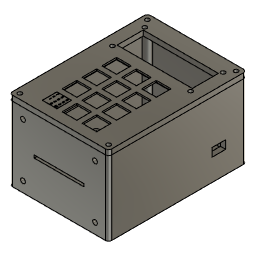
BinaryInterfacer v13 (Autodesk Fusion 360 design; units mm, degrees)
Autodesk Fusion 360 part; units mm, degrees
(part 1 of 2)
sketch "Sketch1" plane through (0, 0, 0) normal (0, 0, 1) x (1, 0, 0) in component "Plate"
  line L0 (6.725, 7.025) -> (-6.725, 7.025)
  line L1 (-7.025, 6.725) -> (-7.025, -6.725)
  line L2 (-6.725, -7.025) -> (6.725, -7.025)
  line L3 (7.025, -6.725) -> (7.025, 6.725)
  line L4 (7.025, 7.025) -> (-7.025, -7.025) construction
  line L5 (-7.025, 7.025) -> (7.025, -7.025) construction
  arc A0 (-6.725, 7.025) -> (-7.025, 6.725) centre (-6.725, 6.725) ccw
  arc A1 (-7.025, -6.725) -> (-6.725, -7.025) centre (-6.725, -6.725) ccw
  arc A2 (6.725, -7.025) -> (7.025, -6.725) centre (6.725, -6.725) ccw
  arc A3 (7.025, 6.725) -> (6.725, 7.025) centre (6.725, 6.725) ccw
  line L6 (26.075, -6.725) -> (26.075, 6.725)
  arc A4 (26.075, 6.725) -> (25.775, 7.025) centre (25.775, 6.725) ccw
  line L7 (25.775, 7.025) -> (12.325, 7.025)
  arc A5 (12.325, 7.025) -> (12.025, 6.725) centre (12.325, 6.725) ccw
  line L8 (12.025, 6.725) -> (12.025, -6.725)
  arc A6 (12.025, -6.725) -> (12.325, -7.025) centre (12.325, -6.725) ccw
  line L9 (12.325, -7.025) -> (25.775, -7.025)
  arc A7 (25.775, -7.025) -> (26.075, -6.725) centre (25.775, -6.725) ccw
  line L10 (45.125, -6.725) -> (45.125, 6.725)
  arc A8 (45.125, 6.725) -> (44.825, 7.025) centre (44.825, 6.725) ccw
  line L11 (44.825, 7.025) -> (31.375, 7.025)
  arc A9 (31.375, 7.025) -> (31.075, 6.725) centre (31.375, 6.725) ccw
  line L12 (31.075, 6.725) -> (31.075, -6.725)
  arc A10 (31.075, -6.725) -> (31.375, -7.025) centre (31.375, -6.725) ccw
  line L13 (31.375, -7.025) -> (44.825, -7.025)
  arc A11 (44.825, -7.025) -> (45.125, -6.725) centre (44.825, -6.725) ccw
  line L14 (7.025, 12.325) -> (7.025, 25.775)
  arc A12 (7.025, 25.775) -> (6.725, 26.075) centre (6.725, 25.775) ccw
  line L15 (6.725, 26.075) -> (-6.725, 26.075)
  arc A13 (-6.725, 26.075) -> (-7.025, 25.775) centre (-6.725, 25.775) ccw
  line L16 (-7.025, 25.775) -> (-7.025, 12.325)
  arc A14 (-7.025, 12.325) -> (-6.725, 12.025) centre (-6.725, 12.325) ccw
  line L17 (-6.725, 12.025) -> (6.725, 12.025)
  arc A15 (6.725, 12.025) -> (7.025, 12.325) centre (6.725, 12.325) ccw
  line L18 (26.075, 12.325) -> (26.075, 25.775)
  arc A16 (26.075, 25.775) -> (25.775, 26.075) centre (25.775, 25.775) ccw
  line L19 (25.775, 26.075) -> (12.325, 26.075)
  arc A17 (12.325, 26.075) -> (12.025, 25.775) centre (12.325, 25.775) ccw
  line L20 (12.025, 25.775) -> (12.025, 12.325)
  arc A18 (12.025, 12.325) -> (12.325, 12.025) centre (12.325, 12.325) ccw
  line L21 (12.325, 12.025) -> (25.775, 12.025)
  arc A19 (25.775, 12.025) -> (26.075, 12.325) centre (25.775, 12.325) ccw
  line L22 (45.125, 12.325) -> (45.125, 25.775)
  arc A20 (45.125, 25.775) -> (44.825, 26.075) centre (44.825, 25.775) ccw
  line L23 (44.825, 26.075) -> (31.375, 26.075)
  arc A21 (31.375, 26.075) -> (31.075, 25.775) centre (31.375, 25.775) ccw
  line L24 (31.075, 25.775) -> (31.075, 12.325)
  arc A22 (31.075, 12.325) -> (31.375, 12.025) centre (31.375, 12.325) ccw
  line L25 (31.375, 12.025) -> (44.825, 12.025)
  arc A23 (44.825, 12.025) -> (45.125, 12.325) centre (44.825, 12.325) ccw
  line L26 (7.025, 31.375) -> (7.025, 44.825)
  arc A24 (7.025, 44.825) -> (6.725, 45.125) centre (6.725, 44.825) ccw
  line L27 (6.725, 45.125) -> (-6.725, 45.125)
  arc A25 (-6.725, 45.125) -> (-7.025, 44.825) centre (-6.725, 44.825) ccw
  line L28 (-7.025, 44.825) -> (-7.025, 31.375)
  arc A26 (-7.025, 31.375) -> (-6.725, 31.075) centre (-6.725, 31.375) ccw
  line L29 (-6.725, 31.075) -> (6.725, 31.075)
  arc A27 (6.725, 31.075) -> (7.025, 31.375) centre (6.725, 31.375) ccw
  line L30 (26.075, 31.375) -> (26.075, 44.825)
  arc A28 (26.075, 44.825) -> (25.775, 45.125) centre (25.775, 44.825) ccw
  line L31 (25.775, 45.125) -> (12.325, 45.125)
  arc A29 (12.325, 45.125) -> (12.025, 44.825) centre (12.325, 44.825) ccw
  line L32 (12.025, 44.825) -> (12.025, 31.375)
  arc A30 (12.025, 31.375) -> (12.325, 31.075) centre (12.325, 31.375) ccw
  line L33 (12.325, 31.075) -> (25.775, 31.075)
  arc A31 (25.775, 31.075) -> (26.075, 31.375) centre (25.775, 31.375) ccw
  line L34 (45.125, 31.375) -> (45.125, 44.825)
  arc A32 (45.125, 44.825) -> (44.825, 45.125) centre (44.825, 44.825) ccw
  line L35 (44.825, 45.125) -> (31.375, 45.125)
  arc A33 (31.375, 45.125) -> (31.075, 44.825) centre (31.375, 44.825) ccw
  line L36 (31.075, 44.825) -> (31.075, 31.375)
  arc A34 (31.075, 31.375) -> (31.375, 31.075) centre (31.375, 31.375) ccw
  line L37 (31.375, 31.075) -> (44.825, 31.075)
  arc A35 (44.825, 31.075) -> (45.125, 31.375) centre (44.825, 31.375) ccw
  arc A36 (12.025, -25.775) -> (12.325, -26.075) centre (12.325, -25.775) ccw
  arc A37 (25.775, -26.075) -> (26.075, -25.775) centre (25.775, -25.775) ccw
  arc A38 (26.075, -12.325) -> (25.775, -12.025) centre (25.775, -12.325) ccw
  arc A39 (12.325, -12.025) -> (12.025, -12.325) centre (12.325, -12.325) ccw
  line L38 (12.325, -26.075) -> (25.775, -26.075)
  line L39 (26.075, -25.775) -> (26.075, -12.325)
  line L40 (12.025, -12.325) -> (12.025, -25.775)
  line L41 (25.775, -12.025) -> (12.325, -12.025)
  line L42 (-28.45, 96.125) -> (66.55, 96.125)
  line L43 (66.55, 96.125) -> (66.55, -36.075)
  line L44 (66.55, -36.075) -> (-28.45, -36.075)
  line L45 (-28.45, -36.075) -> (-28.45, 96.125)
  line L46 (26.075, -19.05) -> (66.55, -19.05) construction
  line L47 (12.025, -19.05) -> (-28.45, -19.05) construction
  line L48 (19.05, 96.125) -> (19.05, -36.075) construction
  line L49 (59.05, 50.125) -> (-20.95, 50.125)
  line L50 (-20.95, 50.125) -> (-20.95, 86.125)
  line L51 (-20.95, 86.125) -> (59.05, 86.125)
  line L52 (59.05, 86.125) -> (59.05, 50.125)
  line L53 (59.05, 50.125) -> (-20.95, 86.125) construction
  line L54 (-20.95, 50.125) -> (59.05, 86.125) construction
  line L55 (-16.95, 80.625) -> (55.05, 80.625)
  line L56 (55.05, 80.625) -> (55.05, 55.625)
  line L57 (55.05, 55.625) -> (-16.95, 55.625)
  line L58 (-16.95, 55.625) -> (-16.95, 80.625)
  line L59 (-16.95, 80.625) -> (55.05, 55.625) construction
  line L60 (55.05, 80.625) -> (-16.95, 55.625) construction
  line L61 (-18.45, 86.125) -> (-18.45, 50.125) construction
  line L62 (56.55, 86.125) -> (56.55, 50.125) construction
  line L63 (-18.45, 68.125) -> (-20.95, 68.125) construction
  line L64 (56.55, 68.125) -> (59.05, 68.125) construction
  circle A40 centre (-18.45, 83.625) radius 2
  circle A41 centre (-18.45, 52.625) radius 2
  circle A42 centre (56.55, 83.625) radius 2
  circle A43 centre (56.55, 52.625) radius 2
  circle A44 centre (-23.45, -31.075) radius 5 construction
  circle A45 centre (-23.45, -31.075) radius 2
  circle A46 centre (61.55, -31.075) radius 2
  line L65 (19.05, 30.025) -> (23, 30.025) construction
  circle A47 centre (-23.45, 91.125) radius 2
  circle A48 centre (61.55, 91.125) radius 2
  line L66 (-10.025, 48.125) -> (48.125, 48.125)
  line L67 (48.125, 48.125) -> (48.125, -29.075)
  line L68 (48.125, -29.075) -> (-10.025, -29.075)
  line L69 (-10.025, -29.075) -> (-10.025, 48.125)
  line L70 (-7.025, 38.1) -> (-10.025, 38.1) construction
  line L71 (45.125, 38.1) -> (48.125, 38.1) construction
  line L72 (19.05, 45.125) -> (19.05, 48.125) construction
  line L73 (19.05, -26.075) -> (19.05, -29.075) construction
  arc A49 (31.075, -25.775) -> (31.375, -26.075) centre (31.375, -25.775) ccw
  line L74 (31.375, -26.075) -> (44.825, -26.075)
  line L75 (44.825, -12.025) -> (31.375, -12.025)
  line L76 (45.125, -25.775) -> (45.125, -12.325)
  line L77 (31.075, -12.325) -> (31.075, -25.775)
  arc A50 (45.125, -12.325) -> (44.825, -12.025) centre (44.825, -12.325) ccw
  arc A51 (44.825, -26.075) -> (45.125, -25.775) centre (44.825, -25.775) ccw
  arc A52 (31.375, -12.025) -> (31.075, -12.325) centre (31.375, -12.325) ccw
  line L78 (7.025, -25.775) -> (7.025, -12.325)
  arc A53 (6.725, -26.075) -> (7.025, -25.775) centre (6.725, -25.775) ccw
  line L79 (-6.725, -26.075) -> (6.725, -26.075)
  arc A54 (-7.025, -25.775) -> (-6.725, -26.075) centre (-6.725, -25.775) ccw
  line L80 (-7.025, -12.325) -> (-7.025, -25.775)
  line L81 (6.725, -12.025) -> (-6.725, -12.025)
  arc A55 (-6.725, -12.025) -> (-7.025, -12.325) centre (-6.725, -12.325) ccw
  arc A56 (7.025, -12.325) -> (6.725, -12.025) centre (6.725, -12.325) ccw
  line L82 (-10.025, -9.025) -> (10.025, -9.025)
  line L83 (10.025, -9.025) -> (10.025, -29.075)
  line L84 (6.725, -12.025) -> (6.725, -9.025) construction
  line L85 (7.025, -12.325) -> (10.025, -12.325) construction
  point P0 (19.05, 68.125)
  point P1 (19.05, 68.125)
  dimension "d1" = 14.05
  dimension "d2" = 14.05
  dimension "d3" = 0.3
  dimension "d6" = 19.05
  dimension "d7" = 19.05
  dimension "d14" = 0
  dimension "d15" = -19.05
  dimension "d24" = 95
  dimension "d25" = 10
  dimension "d26" = 80
  dimension "d27" = 36
  dimension "d29" = 72
  dimension "d30" = 25
  dimension "d31" = 75
  dimension "d32" = 4
  dimension "d33" = 2.5
  dimension "d34" = 31
  dimension "d35" = 10
  dimension "d36" = 5
  dimension "d37" = 10
  dimension "d38" = 3
  constraint horizontal L0
  constraint perpendicular L0 L1
  constraint parallel L0 L2
  constraint parallel L1 L3
  constraint coincident L4 origin
  constraint coincident L5 origin
  constraint coincident L5.start L0
  constraint coincident L5.start L1
  constraint tangent L0 A0
  constraint tangent L1 A0
  constraint coincident L4.end L2
  constraint coincident L4.end L1
  constraint tangent L2 A1
  constraint tangent L1 A1
  constraint equal A0 A1
  constraint coincident L5.end L2
  constraint coincident L5.end L3
  constraint tangent L2 A2
  constraint tangent L3 A2
  constraint equal A0 A2
  constraint coincident L4.start L3
  constraint coincident L4.start L0
  constraint tangent L3 A3
  constraint tangent L0 A3
  constraint equal A0 A3
  constraint horizontal L42
  constraint vertical L43
  constraint horizontal L44
  constraint vertical L45
  constraint midpoint L39 L46.start
  constraint coincident L43 L46.end
  constraint perpendicular L43 L46
  constraint midpoint L40 L47.start
  constraint coincident L45 L47.end
  constraint perpendicular L45 L47
  constraint equal L46 L47
  constraint midpoint L42 L48.start
  constraint midpoint L44 L48.end
  constraint horizontal L49
  constraint perpendicular L49 L50
  constraint parallel L49 L51
  constraint parallel L50 L52
  constraint coincident L53 P1
  constraint coincident L54 P1
  constraint horizontal L55
  constraint perpendicular L55 L56
  constraint parallel L55 L57
  constraint parallel L56 L58
  constraint coincident L59 P1
  constraint coincident L60 P1
  constraint coincident P1 P0
  constraint coincident L51 L61.start
  constraint coincident L49 L61.end
  constraint perpendicular L49 L61
  constraint coincident L51 L62.start
  constraint coincident L49 L62.end
  constraint perpendicular L49 L62
  constraint midpoint L61 L63.start
  constraint midpoint L50 L63.end
  constraint midpoint L62 L64.start
  constraint midpoint L52 L64.end
  constraint equal L63 L64
  constraint coincident L61 A40.centre
  constraint coincident L61 A41.centre
  constraint coincident L48 P1
  constraint symmetric L48 A40 A42
  constraint symmetric L48 A41 A43
  constraint equal A42 A43
  constraint tangent L44 A44
  constraint tangent L45 A44
  constraint concentric A44 A45
  constraint equal A40 A45
  constraint symmetric L48 A45 A46
  constraint midpoint L48 L65.start
  constraint perpendicular L48 L65
  constraint symmetric A45 L65 A47
  constraint symmetric A46 L65 A48
  constraint horizontal L66
  constraint vertical L67
  constraint horizontal L68
  constraint vertical L69
  constraint midpoint L28 L70.start
  constraint coincident L69 L70.end
  constraint perpendicular L69 L70
  constraint midpoint L34 L71.start
  constraint coincident L67 L71.end
  constraint perpendicular L67 L71
  constraint coincident L31 L72.start
  constraint coincident L66 L72.end
  constraint perpendicular L66 L72
  constraint coincident L38 L73.start
  constraint coincident L68 L73.end
  constraint perpendicular L68 L73
  constraint equal L71 L73
  constraint equal L71 L72
  constraint equal L70 L72
  constraint coincident L48 L72.end
  constraint coincident L48 L73.end
  constraint coincident L69 L82.start
  constraint perpendicular L69 L82
  constraint coincident L68 L83.end
  constraint perpendicular L68 L83
  constraint coincident L82 L84.end
  constraint perpendicular L82 L84
  constraint coincident L83 L85.end
  constraint perpendicular L83 L85
  constraint equal L84 L85
  constraint equal L70 L84
  measures "d1" distance of L4.end L5.end
  measures "d2" distance of L5.start L4.end
  measures "d3" radius of A0
  measures "d24" distance of L43.end L44.end
  measures "d25" distance of L38 L44
  measures "d26" distance of L50.end L51.end
  measures "d27" distance of L49.end L50.end
  measures "d29" distance of L56.end L57.end
  measures "d30" distance of L55.end L56.end
  measures "d31" distance of L61 L62
  measures "d32" diameter of A40
  measures "d33" distance of L51 A40.centre
  measures "d34" distance of A40.centre A41.centre
  measures "d35" distance of L42 L51
  measures "d36" distance of L35 L49
  measures "d37" diameter of A44
  measures "d38" distance of L70.start L70.end
extrude "Extrude1" add sketch "Sketch1" against normal blind 1.5 contours L66 L67 L68 L69 L82 L83 | L68 L69 L82 L83 makes body 1 in component "Plate"
extrude "Extrude2" add sketch "Sketch1" against normal blind 5 contours L42 L43 L44 L45 | L49 L50 L51 L52 | L68 L69 L82 L83 | L78 A53 L79 A54 L80 L81 A55 A56 bodies 1 in component "Plate"
extrude "Extrude4" cut sketch "Sketch1" against normal blind 3 contours L78 A53 L79 A54 L80 L81 A55 A56 bodies 1 in component "Plate"
fillet "Fillet1" radius 3 4 edges at (-28.45, -36.075, -2.5) (66.55, -36.075, -2.5) (-28.45, 96.125, -2.5) (66.55, 96.125, -2.5) on bodies 1 in component "Plate"
sketch "Sketch1 (2)" plane through (0, 0, -3) normal (0, 0, 1) x (-1, 0, 0) in component "Insert"
  arc A0 (-7.025, 12.325) -> (-6.725, 12.025) centre (-6.725, 12.325) ccw
  line L0 (-6.725, 12.025) -> (6.725, 12.025)
  arc A1 (6.725, 12.025) -> (7.025, 12.325) centre (6.725, 12.325) ccw
  line L1 (7.025, 12.325) -> (7.025, 25.775)
  arc A2 (7.025, 25.775) -> (6.725, 26.075) centre (6.725, 25.775) ccw
  line L2 (6.725, 26.075) -> (-6.725, 26.075)
  arc A3 (-6.725, 26.075) -> (-7.025, 25.775) centre (-6.725, 25.775) ccw
  line L3 (-7.025, 25.775) -> (-7.025, 12.325)
  line L4 (6.925, 12.325) -> (6.925, 25.775)
  arc A4 (6.925, 25.775) -> (6.725, 25.975) centre (6.725, 25.775) ccw
  line L5 (6.725, 25.975) -> (-6.725, 25.975)
  arc A5 (-6.725, 25.975) -> (-6.925, 25.775) centre (-6.725, 25.775) ccw
  line L6 (-6.925, 25.775) -> (-6.925, 12.325)
  arc A6 (-6.925, 12.325) -> (-6.725, 12.125) centre (-6.725, 12.325) ccw
  line L7 (-6.725, 12.125) -> (6.725, 12.125)
  arc A7 (6.725, 12.125) -> (6.925, 12.325) centre (6.725, 12.325) ccw
  dimension "d47" = -0.1
extrude "Extrude1'" add sketch "Sketch1 (2)" along normal blind 3 separate body contours L4 A4 L5 A5 L6 A6 L7 A7 makes body 2 in component "Insert"
sketch "Sketch2" plane through (0, 0, 0) normal (0, 0, 1) x (-1, 0, 0) in component "Insert"
  arc A0 (6.725, 12.125) -> (6.925, 12.325) centre (6.725, 12.325) ccw
  line L0 (6.925, 12.325) -> (6.925, 25.775)
  arc A1 (6.925, 25.775) -> (6.725, 25.975) centre (6.725, 25.775) ccw
  line L1 (6.725, 25.975) -> (-6.725, 25.975)
  arc A2 (-6.725, 25.975) -> (-6.925, 25.775) centre (-6.725, 25.775) ccw
  line L2 (-6.925, 25.775) -> (-6.925, 12.325)
  arc A3 (-6.925, 12.325) -> (-6.725, 12.125) centre (-6.725, 12.325) ccw
  line L3 (-6.725, 12.125) -> (6.725, 12.125)
  line L4 (2.3083, 12.125) -> (2.3083, 25.975) construction
  line L5 (-2.3083, 25.975) -> (-2.3083, 12.125) construction
  line L6 (2.3083, 19.05) -> (6.925, 19.05) construction
  line L7 (2.3083, 19.05) -> (-2.3083, 19.05) construction
  line L8 (-2.3083, 19.05) -> (-6.925, 19.05) construction
  line L9 (-6.925, 15.5875) -> (6.925, 15.5875) construction
  line L10 (6.925, 19.05) -> (-6.925, 19.05) construction
  line L11 (-6.925, 22.5125) -> (6.925, 22.5125) construction
  line L12 (0, 12.125) -> (0, 15.5875) construction
  line L13 (0, 15.5875) -> (0, 19.05) construction
  line L14 (0, 19.05) -> (0, 22.5125) construction
  line L15 (0, 22.5125) -> (0, 25.975) construction
  line L16 (4.6167, 13.8563) -> (-4.6167, 13.8563) construction
  line L17 (-4.6167, 13.8563) -> (-4.6167, 24.2438) construction
  line L18 (-4.6167, 24.2438) -> (4.6167, 24.2438) construction
  line L19 (4.6167, 24.2438) -> (4.6167, 13.8563) construction
  line L20 (1, 26.2438) -> (-1, 26.2438) construction
  line L21 (-1, 26.2438) -> (-1, 22.2437) construction
  line L22 (-1, 22.2437) -> (1, 22.2438) construction
  line L23 (1, 22.2438) -> (1, 26.2438) construction
  line L24 (1, 22.2438) -> (-1, 26.2438) construction
  line L25 (1, 26.2438) -> (-1, 22.2437) construction
  line L26 (5.6167, 26.2437) -> (3.6167, 22.2437) construction
  line L27 (5.6167, 26.2437) -> (3.6167, 26.2438) construction
  line L28 (3.6167, 26.2438) -> (3.6167, 22.2437) construction
  line L29 (3.6167, 22.2437) -> (5.6167, 22.2437) construction
  line L30 (5.6167, 22.2437) -> (5.6167, 26.2437) construction
  line L31 (5.6167, 22.2437) -> (3.6167, 26.2438) construction
  line L32 (-3.6167, 19.3188) -> (-5.6167, 15.3187) construction
  line L33 (-3.6167, 19.3188) -> (-5.6167, 19.3188) construction
  line L34 (-5.6167, 19.3188) -> (-5.6167, 15.3187) construction
  line L35 (-5.6167, 15.3187) -> (-3.6167, 15.3188) construction
  line L36 (-3.6167, 15.3188) -> (-3.6167, 19.3188) construction
  line L37 (5.6167, 19.3187) -> (3.6167, 19.3188) construction
  line L38 (3.6167, 19.3188) -> (3.6167, 15.3187) construction
  line L39 (3.6167, 15.3187) -> (5.6167, 15.3187) construction
  line L40 (5.6167, 15.3187) -> (5.6167, 19.3187) construction
  line L41 (5.6167, 19.3187) -> (3.6167, 15.3187) construction
  line L42 (-3.6167, 15.3188) -> (-5.6167, 19.3188) construction
  line L43 (5.6167, 15.3187) -> (3.6167, 19.3188) construction
  line L44 (1, 15.8563) -> (-1, 15.8563) construction
  line L45 (-1, 15.8563) -> (-1, 11.8562) construction
  line L46 (-1, 11.8562) -> (1, 11.8563) construction
  line L47 (1, 11.8563) -> (1, 15.8563) construction
  line L48 (-3.6167, 15.8562) -> (-5.6167, 15.8563) construction
  line L49 (-5.6167, 15.8563) -> (-5.6167, 11.8562) construction
  line L50 (-5.6167, 11.8562) -> (-3.6167, 11.8562) construction
  line L51 (-3.6167, 11.8562) -> (-3.6167, 15.8562) construction
  line L52 (-3.6167, 26.2437) -> (-5.6167, 26.2438) construction
  line L53 (-5.6167, 26.2438) -> (-5.6167, 22.2437) construction
  line L54 (-5.6167, 22.2437) -> (-3.6167, 22.2437) construction
  line L55 (-3.6167, 22.2437) -> (-3.6167, 26.2437) construction
  line L56 (5.6167, 15.8562) -> (3.6167, 15.8563) construction
  line L57 (3.6167, 15.8563) -> (3.6167, 11.8562) construction
  line L58 (3.6167, 11.8562) -> (5.6167, 11.8562) construction
  line L59 (5.6167, 11.8562) -> (5.6167, 15.8562) construction
  line L60 (5.6167, 11.8562) -> (3.6167, 15.8563) construction
  line L61 (1, 15.8563) -> (-1, 11.8562) construction
  line L62 (-3.6167, 22.2437) -> (-5.6167, 26.2438) construction
  line L63 (-3.6167, 26.2437) -> (-5.6167, 22.2437) construction
  line L64 (-3.6167, 11.8562) -> (-5.6167, 15.8563) construction
  line L65 (-3.6167, 15.8562) -> (-5.6167, 11.8562) construction
  line L66 (1, 11.8563) -> (-1, 15.8563) construction
  line L67 (5.6167, 15.8562) -> (3.6167, 11.8562) construction
  line L68 (42.1174, 51.0238) -> (40.1174, 47.0238) construction
  line L69 (46.6174, 51.0238) -> (44.6174, 47.0238) construction
  line L70 (-3.6167, 22.7813) -> (-5.6167, 18.7812) construction
  line L71 (42.1174, 51.0238) -> (40.1174, 51.0238) construction
  line L72 (40.1174, 51.0238) -> (40.1174, 47.0238) construction
  line L73 (40.1174, 47.0238) -> (42.1174, 47.0238) construction
  line L74 (42.1174, 47.0238) -> (42.1174, 51.0238) construction
  line L75 (1, 22.7812) -> (-1, 18.7812) construction
  line L76 (42.1174, 47.0238) -> (40.1174, 51.0238) construction
  line L77 (5.6167, 22.7813) -> (3.6167, 18.7812) construction
  line L78 (46.6174, 51.0238) -> (44.6174, 51.0238) construction
  line L79 (44.6174, 51.0238) -> (44.6174, 47.0238) construction
  line L80 (44.6174, 47.0238) -> (46.6174, 47.0238) construction
  line L81 (46.6174, 47.0238) -> (46.6174, 51.0238) construction
  line L82 (1, 19.3188) -> (-1, 15.3187) construction
  line L83 (1, 22.7812) -> (-1, 22.7813) construction
  line L84 (-1, 22.7813) -> (-1, 18.7812) construction
  line L85 (-1, 18.7812) -> (1, 18.7812) construction
  line L86 (1, 18.7812) -> (1, 22.7812) construction
  line L87 (53.1174, 51.0238) -> (51.1174, 47.0238) construction
  line L88 (1, 15.3188) -> (-1, 19.3188) construction
  line L89 (-3.6167, 22.7813) -> (-5.6167, 22.7813) construction
  line L90 (-5.6167, 22.7813) -> (-5.6167, 18.7812) construction
  line L91 (-5.6167, 18.7812) -> (-3.6167, 18.7813) construction
  line L92 (-3.6167, 18.7813) -> (-3.6167, 22.7813) construction
  line L93 (53.1174, 51.0238) -> (51.1174, 51.0238) construction
  line L94 (51.1174, 51.0238) -> (51.1174, 47.0238) construction
  line L95 (51.1174, 47.0238) -> (53.1174, 47.0238) construction
  line L96 (53.1174, 47.0238) -> (53.1174, 51.0238) construction
  line L97 (-3.6167, 18.7813) -> (-5.6167, 22.7813) construction
  line L98 (57.6174, 47.0238) -> (55.6174, 51.0238) construction
  line L99 (1, 18.7812) -> (-1, 22.7813) construction
  line L100 (1, 19.3188) -> (-1, 19.3188) construction
  line L101 (-1, 19.3188) -> (-1, 15.3187) construction
  line L102 (-1, 15.3187) -> (1, 15.3188) construction
  line L103 (1, 15.3188) -> (1, 19.3188) construction
  line L104 (57.6174, 51.0238) -> (55.6174, 47.0238) construction
  line L105 (5.6167, 18.7813) -> (3.6167, 22.7813) construction
  line L106 (57.6174, 51.0238) -> (55.6174, 51.0238) construction
  line L107 (55.6174, 51.0238) -> (55.6174, 47.0238) construction
  line L108 (55.6174, 47.0238) -> (57.6174, 47.0238) construction
  line L109 (57.6174, 47.0238) -> (57.6174, 51.0238) construction
  line L110 (53.1174, 47.0238) -> (51.1174, 51.0238) construction
  line L111 (5.6167, 22.7813) -> (3.6167, 22.7813) construction
  line L112 (3.6167, 22.7813) -> (3.6167, 18.7812) construction
  line L113 (3.6167, 18.7812) -> (5.6167, 18.7813) construction
  line L114 (5.6167, 18.7813) -> (5.6167, 22.7813) construction
  line L115 (46.6174, 47.0238) -> (44.6174, 51.0238) construction
  line L116 (0, 20.7812) -> (4.6167, 20.7812) construction
  line L117 (0, 20.7812) -> (-4.6167, 20.7812) construction
  line L118 (0, 17.3188) -> (-4.6167, 17.3188) construction
  line L119 (0, 17.3188) -> (4.6167, 17.3188) construction
  point P0 (4.6167, 19.05)
  point P1 (0, 17.3188)
  point P2 (-4.6167, 19.05)
  point P3 (0, 20.7812)
  point P4 (0, 24.2438)
  point P5 (0, 13.8563)
  point P6 (4.6167, 13.8563)
  point P7 (-4.6167, 24.2438)
  point P8 (0, 24.2438)
  point P9 (4.6167, 24.2438)
  point P10 (-4.6167, 17.3188)
  point P11 (4.6167, 17.3188)
  point P12 (-4.6167, 13.8563)
  point P13 (0, 13.8563)
  point P14 (0, 17.3188)
  point P15 (4.6167, 20.7812)
  point P16 (0, 20.7812)
  point P17 (-4.6167, 20.7812)
  point P18 (56.6174, 49.0238)
  point P19 (52.1174, 49.0238)
  point P20 (45.6174, 49.0238)
  point P21 (41.1174, 49.0238)
  dimension "d50" = 2
  dimension "d51" = 2
  dimension "d52" = 4
  dimension "d53" = 2
  dimension "d54" = 2
  dimension "d55" = 4
  dimension "d56" = 2
  dimension "d57" = 2
  dimension "d58" = 2
  dimension "d59" = 4
  dimension "d60" = 2
  dimension "d61" = 4
  dimension "d62" = 2
  dimension "d63" = 2
  dimension "d64" = 2
  dimension "d65" = 2
  dimension "d66" = 2
  dimension "d67" = 4
  dimension "d68" = 2
  dimension "d69" = 4
  dimension "d70" = 2
  dimension "d71" = 4
  dimension "d72" = 2
  dimension "d73" = 4
  dimension "d74" = 2
  dimension "d75" = 2
  dimension "d76" = 2
  dimension "d77" = 2
  dimension "d78" = 2
  dimension "d79" = 2
  dimension "d80" = 2
  dimension "d81" = 2
  dimension "d82" = 2
  dimension "d83" = 4
  dimension "d84" = 2
  dimension "d85" = 4
  dimension "d86" = 2
  dimension "d87" = 4
  dimension "d88" = 2
  dimension "d89" = 4
  dimension "d90" = 2
  dimension "d91" = 4
  dimension "d92" = 2
  dimension "d93" = 4
  dimension "d94" = 2
  dimension "d95" = 4
  dimension "d96" = 2
  dimension "d97" = 4
  text T0 "0" font "Arial" height 2 align centre middle in box 2 x 4 at (1, 26.2438) x (-1, 0) y (0, -1) spacing 1 kerned
  text T1 "6" font "Arial" height 2 align centre middle in box 2 x 4 at (-3.6167, 19.3188) x (-1, 0) y (0, -1) spacing 1 kerned
  text T2 "4" font "Arial" height 2 align centre middle in box 2 x 4 at (5.6167, 19.3187) x (-1, 0) y (0, -1) spacing 1 kerned
  text T3 "8" font "Arial" height 2 align centre middle in box 2 x 4 at (1, 15.8563) x (-1, 0) y (0, -1) spacing 1 kerned
  text T4 "9" font "Arial" height 2 align centre middle in box 2 x 4 at (-3.6167, 15.8562) x (-1, 0) y (0, -1) spacing 1 kerned
  text T5 "M" font "Arial" height 2 align centre middle in box 2 x 4 at (-3.6167, 26.2437) x (-1, 0) y (0, -1) spacing 1 kerned
  text T6 "7" font "Arial" height 2 align centre middle in box 2 x 4 at (5.6167, 15.8562) x (-1, 0) y (0, -1) spacing 1 kerned
  text T7 "2" font "Arial" height 2 align centre middle in box 2 x 4 at (1, 22.7812) x (-1, 0) y (0, -1) spacing 1 kerned
  text T8 "3" font "Arial" height 2 align centre middle in box 2 x 4 at (-3.6167, 22.7813) x (-1, 0) y (0, -1) spacing 1 kerned
  text T9 "5" font "Arial" height 2 align centre middle in box 2 x 4 at (1, 19.3188) x (-1, 0) y (0, -1) spacing 1 kerned
  text T10 "1" font "Arial" height 2 align centre middle in box 2 x 4 at (5.6167, 22.7813) x (-1, 0) y (0, -1) spacing 1 kerned
  constraint coincident L3 L4.start
  constraint coincident L1 L4.end
  constraint perpendicular L1 L4
  constraint coincident L1 L5.start
  constraint coincident L3 L5.end
  constraint perpendicular L3 L5
  constraint midpoint L4 L6.start
  constraint midpoint L0 L6.end
  constraint midpoint L5 L7.end
  constraint midpoint L2 L8.end
  constraint equal L7 L8
  constraint equal L6 L7
  constraint coincident L2 L9.start
  constraint coincident L0 L9.end
  constraint perpendicular L0 L9
  constraint coincident L0 L6.end
  constraint coincident L2 L8.end
  constraint perpendicular L2 L10
  constraint coincident L2 L11.start
  constraint coincident L0 L11.end
  constraint perpendicular L0 L11
  constraint midpoint L3 L12.start
  constraint midpoint L9 L12.end
  constraint midpoint L10 L13.end
  constraint midpoint L11 L14.end
  constraint midpoint L1 L15.end
  constraint equal L13 L14
  constraint equal L12 L13
  constraint equal L12 L15
  constraint midpoint L6 P0
  constraint midpoint L13 P14
  constraint midpoint L8 P2
  constraint midpoint L14 P16
  constraint midpoint L15 P8
  constraint midpoint L12 P13
  constraint horizontal L16
  constraint vertical L17
  constraint horizontal L18
  constraint vertical L19
  constraint coincident P13 L16
  constraint coincident P0 L19
  constraint coincident P8 L18
  constraint coincident P2 L17
  constraint vertical L21
  constraint coincident L22.end
  constraint coincident L20.end
  constraint coincident L20.start
  constraint coincident L21.end
  constraint vertical L28
  constraint coincident L29.end
  constraint coincident L27.end
  constraint coincident L26.start
  constraint coincident L26.end
  constraint vertical L38
  constraint coincident L39.end
  constraint coincident L37.end
  constraint coincident L37.start
  constraint coincident L38.end
  constraint vertical L34
  constraint coincident L35.end
  constraint coincident L33.end
  constraint coincident L32.start
  constraint coincident L32.end
  constraint vertical L57
  constraint coincident L58.end
  constraint coincident L56.end
  constraint coincident L56.start
  constraint coincident L57.end
  constraint vertical L53
  constraint coincident L54.end
  constraint coincident L52.end
  constraint coincident L52.start
  constraint coincident L53.end
  constraint vertical L45
  constraint coincident L46.end
  constraint coincident L44.end
  constraint coincident L44.start
  constraint coincident L45.end
  constraint vertical L49
  constraint coincident L50.end
  constraint coincident L48.end
  constraint coincident L48.start
  constraint coincident L49.end
  constraint vertical L84
  constraint coincident L85.end
  constraint coincident L83.end
  constraint coincident L75.start
  constraint coincident L75.end
  constraint vertical L90
  constraint coincident L91.end
  constraint coincident L89.end
  constraint coincident L70.start
  constraint coincident L70.end
  constraint vertical L94
  constraint coincident L95.end
  constraint coincident L93.end
  constraint coincident L87.start
  constraint coincident L87.end
  constraint vertical L107
  constraint coincident L98.start
  constraint coincident L98.end
  constraint coincident L104.start
  constraint coincident L104.end
  constraint vertical L101
  constraint coincident L88.start
  constraint coincident L88.end
  constraint coincident L82.start
  constraint coincident L82.end
  constraint vertical L112
  constraint coincident L105.start
  constraint coincident L105.end
  constraint coincident L77.start
  constraint coincident L77.end
  constraint vertical L72
  constraint coincident L73.end
  constraint coincident L71.end
  constraint coincident L68.start
  constraint coincident L68.end
  constraint vertical L79
  constraint coincident L80.end
  constraint coincident L78.end
  constraint coincident L69.start
  constraint coincident L69.end
  constraint midpoint L60 P6
  constraint midpoint L62 P7
  constraint coincident P8
  constraint midpoint L31 P9
  constraint midpoint L32 P10
  constraint midpoint L43 P11
  constraint midpoint L64 P12
  constraint midpoint L61 P13
  constraint midpoint L82 P14
  constraint midpoint L77 P15
  constraint midpoint L99 P16
  constraint midpoint L70 P17
  constraint midpoint L104 P18
  constraint midpoint L110 P19
  constraint midpoint L115 P20
  constraint midpoint L68 P21
  constraint coincident P9 L18.end
  constraint coincident P8 P4
  constraint coincident P7 L17.end
  constraint coincident P6 L16.start
  constraint coincident P13 P5
  constraint coincident P12 L16.end
  constraint coincident P16 P3
  constraint coincident L19 P15
  constraint perpendicular L19 L116
  constraint coincident L17 P17
  constraint perpendicular L17 L117
  constraint coincident P14 P1
  constraint coincident L17 P10
  constraint perpendicular L17 L118
  constraint coincident L19 P11
  constraint perpendicular L19 L119
  constraint coincident P11 L119.end
  constraint coincident P10 L118.end
  constraint coincident P15 L116.end
  constraint coincident P17 L117.end
extrude "Extrude2'" cut sketch "Sketch2" against normal blind 0.1 text T6 T3 T4 T1 T9 T2 T10 T7 T8 T5 T0 bodies 2 in component "Insert"
sketch "Sketch4" plane through (0, 0, 0) normal (0, 0, 1) x (-1, 0, 0) in component "Insert"
  line L0 (-3.9175, 23.5412) -> (-3.9175, 25.2438)
  line L1 (-3.9175, 25.2438) -> (-3.6624, 25.2438)
  line L2 (-3.6624, 25.2438) -> (-3.6624, 23.2438)
  line L3 (-3.6624, 23.2438) -> (-4.0607, 23.2438)
  line L4 (-4.0607, 23.2438) -> (-4.5341, 24.6598)
  spline S0 degree 3 poles (-4.5341, 24.6598) (-4.5532, 24.7174) (-4.5857, 24.8159) (-4.6168, 24.9148) (-4.6296, 24.9559) knots 0 0 0 0 0.018195 0.031107 0.031107 0.031107 0.031107
  spline S1 degree 3 poles (-4.6296, 24.9559) (-4.6441, 24.9109) (-4.6785, 24.8037) (-4.7149, 24.6972) (-4.736, 24.6353) knots 0 0 0 0 0.014162 0.03378 0.03378 0.03378 0.03378
  line L5 (-4.736, 24.6353) -> (-5.2149, 23.2438)
  line L6 (-5.2149, 23.2438) -> (-5.571, 23.2438)
  line L7 (-5.571, 23.2438) -> (-5.571, 25.2438)
  line L8 (-5.571, 25.2438) -> (-5.3158, 25.2438)
  line L9 (-5.3158, 25.2438) -> (-5.3158, 23.5698)
  line L10 (-5.3158, 23.5698) -> (-4.7347, 25.2438)
  line L11 (-4.7347, 25.2438) -> (-4.4959, 25.2438)
  line L12 (-4.4959, 25.2438) -> (-3.9175, 23.5412)
  spline S2 degree 3 poles (0.2149, 21.4122) (0.2346, 21.4338) (0.2726, 21.4755) (0.3036, 21.5226) (0.3186, 21.5452) knots 0 0 0 0 0.008766 0.016888 0.016888 0.016888 0.016888
  line L13 (0.3186, 21.5452) -> (-0.6623, 21.5452)
  line L14 (-0.6623, 21.5452) -> (-0.6623, 21.7813)
  line L15 (-0.6623, 21.7813) -> (0.6596, 21.7813)
  spline S3 degree 3 poles (0.6596, 21.7813) (0.6591, 21.752) (0.6581, 21.6937) (0.64, 21.6383) (0.631, 21.6107) knots 0 0 0 0 0.008716 0.017379 0.017379 0.017379 0.017379
  spline S4 degree 3 poles (0.631, 21.6107) (0.6108, 21.565) (0.5687, 21.4692) (0.5034, 21.3874) (0.4693, 21.3447) knots 0 0 0 0 0.014925 0.031247 0.031247 0.031247 0.031247
  spline S5 degree 3 poles (0.4693, 21.3447) (0.4249, 21.2967) (0.3247, 21.1885) (0.2112, 21.0943) (0.148, 21.0418) knots 0 0 0 0 0.019599 0.044195 0.044195 0.044195 0.044195
  spline S6 degree 3 poles (0.148, 21.0418) (0.0541, 20.9648) (-0.1041, 20.8351) (-0.2381, 20.6809) (-0.2926, 20.6182) knots 0 0 0 0 0.036337 0.061217 0.061217 0.061217 0.061217
  spline S7 degree 3 poles (-0.2926, 20.6182) (-0.326, 20.5693) (-0.3873, 20.4794) (-0.401, 20.3719) (-0.4072, 20.3229) knots 0 0 0 0 0.017457 0.032082 0.032082 0.032082 0.032082
  spline S8 degree 3 poles (-0.4072, 20.3229) (-0.4029, 20.2761) (-0.3943, 20.1829) (-0.3333, 20.112) (-0.3029, 20.0766) knots 0 0 0 0 0.013706 0.027345 0.027345 0.027345 0.027345
  spline S9 degree 3 poles (-0.3029, 20.0766) (-0.2644, 20.0474) (-0.1841, 19.9864) (-0.0832, 19.9798) (-0.0307, 19.9763) knots 0 0 0 0 0.014181 0.029581 0.029581 0.029581 0.029581
  spline S10 degree 3 poles (-0.0307, 19.9763) (0.0246, 19.9799) (0.1302, 19.9867) (0.2134, 20.0517) (0.2531, 20.0828) knots 0 0 0 0 0.016182 0.030941 0.030941 0.030941 0.030941
  spline S11 degree 3 poles (0.2531, 20.0828) (0.2841, 20.1234) (0.3504, 20.2101) (0.3572, 20.3194) (0.3608, 20.3774) knots 0 0 0 0 0.015007 0.032013 0.032013 0.032013 0.032013
  line L16 (0.3608, 20.3774) -> (0.6132, 20.3515)
  spline S12 degree 3 poles (0.6132, 20.3515) (0.6006, 20.2648) (0.577, 20.102) (0.4688, 19.9787) (0.4181, 19.9211) knots 0 0 0 0 0.025635 0.048167 0.048167 0.048167 0.048167
  spline S13 degree 3 poles (0.4181, 19.9211) (0.3542, 19.878) (0.2173, 19.7857) (0.0519, 19.7775) (-0.0362, 19.7731) knots 0 0 0 0 0.022714 0.048594 0.048594 0.048594 0.048594
  spline S14 degree 3 poles (-0.0362, 19.7731) (-0.1252, 19.778) (-0.293, 19.7872) (-0.4283, 19.8862) (-0.4918, 19.9327) knots 0 0 0 0 0.026091 0.049213 0.049213 0.049213 0.049213
  spline S15 degree 3 poles (-0.4918, 19.9327) (-0.5408, 19.9893) (-0.6392, 20.1031) (-0.6528, 20.253) (-0.6596, 20.3283) knots 0 0 0 0 0.021858 0.043952 0.043952 0.043952 0.043952
  spline S16 degree 3 poles (-0.6596, 20.3283) (-0.6575, 20.3684) (-0.6531, 20.4496) (-0.6248, 20.5258) (-0.6105, 20.5643) knots 0 0 0 0 0.011966 0.024231 0.024231 0.024231 0.024231
  spline S17 degree 3 poles (-0.6105, 20.5643) (-0.5901, 20.6049) (-0.5459, 20.693) (-0.482, 20.7681) (-0.4475, 20.8085) knots 0 0 0 0 0.013577 0.029457 0.029457 0.029457 0.029457
  spline S18 degree 3 poles (-0.4475, 20.8085) (-0.3976, 20.8599) (-0.2775, 20.9838) (-0.1459, 21.0953) (-0.0689, 21.1605) knots 0 0 0 0 0.021476 0.051719 0.051719 0.051719 0.051719
  spline S19 degree 3 poles (-0.0689, 21.1605) (-0.0077, 21.2116) (0.0895, 21.2926) (0.181, 21.3799) (0.2149, 21.4122) knots 0 0 0 0 0.023909 0.03794 0.03794 0.03794 0.03794
  line L17 (4.1951, 17.8399) -> (4.1951, 18.3188)
  line L18 (4.1951, 18.3188) -> (4.4407, 18.3188)
  line L19 (4.4407, 18.3188) -> (4.4407, 17.8399)
  line L20 (4.4407, 17.8399) -> (5.3083, 17.8399)
  line L21 (5.3083, 17.8399) -> (5.3083, 17.6148)
  line L22 (5.3083, 17.6148) -> (4.3957, 16.3188)
  line L23 (4.3957, 16.3188) -> (4.1951, 16.3188)
  line L24 (4.1951, 16.3188) -> (4.1951, 17.6148)
  line L25 (4.1951, 17.6148) -> (3.925, 17.6148)
  line L26 (3.925, 17.6148) -> (3.925, 17.8399)
  line L27 (3.925, 17.8399) -> (4.1951, 17.8399)
  spline S20 degree 3 poles (-4.674, 16.3106) (-4.7478, 16.315) (-4.8893, 16.3236) (-5.0053, 16.4043) (-5.0607, 16.4429) knots 0 0 0 0 0.021723 0.041587 0.041587 0.041587 0.041587
  spline S21 degree 3 poles (-5.0607, 16.4429) (-5.1061, 16.4928) (-5.2011, 16.5971) (-5.2276, 16.736) (-5.2415, 16.8085) knots 0 0 0 0 0.019841 0.041499 0.041499 0.041499 0.041499
  line L28 (-5.2415, 16.8085) -> (-4.9973, 16.8276)
  spline S22 degree 3 poles (-4.9973, 16.8276) (-4.9869, 16.7847) (-4.9686, 16.7089) (-4.9239, 16.6452) (-4.9045, 16.6175) knots 0 0 0 0 0.013095 0.023145 0.023145 0.023145 0.023145
  spline S23 degree 3 poles (-4.9045, 16.6175) (-4.8693, 16.5869) (-4.7988, 16.5255) (-4.7056, 16.5168) (-4.659, 16.5125) knots 0 0 0 0 0.013627 0.027319 0.027319 0.027319 0.027319
  spline S24 degree 3 poles (-4.659, 16.5125) (-4.6213, 16.515) (-4.5472, 16.52) (-4.484, 16.5589) (-4.453, 16.578) knots 0 0 0 0 0.011137 0.021906 0.021906 0.021906 0.021906
  spline S25 degree 3 poles (-4.453, 16.578) (-4.4158, 16.6107) (-4.3374, 16.6799) (-4.2933, 16.7749) (-4.2701, 16.8249) knots 0 0 0 0 0.014687 0.031022 0.031022 0.031022 0.031022
  spline S26 degree 3 poles (-4.2701, 16.8249) (-4.2506, 16.8901) (-4.2054, 17.0406) (-4.2023, 17.1981) (-4.2006, 17.2874) knots 0 0 0 0 0.020325 0.04696 0.04696 0.04696 0.04696
  spline S27 degree 3 poles (-4.2006, 17.2874) (-4.2311, 17.2456) (-4.2903, 17.1645) (-4.376, 17.1122) (-4.4175, 17.0868) knots 0 0 0 0 0.01535 0.029798 0.029798 0.029798 0.029798
  spline S28 degree 3 poles (-4.4175, 17.0868) (-4.4606, 17.0677) (-4.5463, 17.0298) (-4.6398, 17.0241) (-4.6862, 17.0213) knots 0 0 0 0 0.014019 0.027861 0.027861 0.027861 0.027861
  spline S29 degree 3 poles (-4.6862, 17.0213) (-4.7652, 17.029) (-4.9239, 17.0445) (-5.044, 17.1494) (-5.1044, 17.2021) knots 0 0 0 0 0.023177 0.046585 0.046585 0.046585 0.046585
  spline S30 degree 3 poles (-5.1044, 17.2021) (-5.1547, 17.2685) (-5.2593, 17.4064) (-5.2709, 17.5795) (-5.277, 17.6694) knots 0 0 0 0 0.02443 0.050792 0.050792 0.050792 0.050792
  spline S31 degree 3 poles (-5.277, 17.6694) (-5.2737, 17.7307) (-5.2673, 17.8522) (-5.2195, 17.964) (-5.1958, 18.0193) knots 0 0 0 0 0.018275 0.036173 0.036173 0.036173 0.036173
  spline S32 degree 3 poles (-5.1958, 18.0193) (-5.1668, 18.0697) (-5.11, 18.1682) (-5.0178, 18.2345) (-4.9727, 18.2669) knots 0 0 0 0 0.017221 0.033669 0.033669 0.033669 0.033669
  spline S33 degree 3 poles (-4.9727, 18.2669) (-4.9232, 18.292) (-4.822, 18.3432) (-4.7087, 18.3496) (-4.6508, 18.3529) knots 0 0 0 0 0.016458 0.033646 0.033646 0.033646 0.033646
  spline S34 degree 3 poles (-4.6508, 18.3529) (-4.5535, 18.3438) (-4.3606, 18.3258) (-4.2198, 18.1929) (-4.1501, 18.1271) knots 0 0 0 0 0.028431 0.056355 0.056355 0.056355 0.056355
  spline S35 degree 3 poles (-4.1501, 18.1271) (-4.0939, 18.0297) (-3.962, 17.801) (-3.9584, 17.5353) (-3.9564, 17.3829) knots 0 0 0 0 0.033238 0.078027 0.078027 0.078027 0.078027
  spline S36 degree 3 poles (-3.9564, 17.3829) (-3.959, 17.2117) (-3.9635, 16.912) (-4.1084, 16.6515) (-4.1706, 16.5398) knots 0 0 0 0 0.050354 0.088177 0.088177 0.088177 0.088177
  spline S37 degree 3 poles (-4.1706, 16.5398) (-4.2393, 16.4729) (-4.3794, 16.3366) (-4.5745, 16.3193) (-4.674, 16.3106) knots 0 0 0 0 0.027864 0.056847 0.056847 0.056847 0.056847
  spline S38 degree 3 poles (0.6589, 14.2778) (0.6556, 14.2165) (0.6493, 14.0993) (0.5889, 13.999) (0.56, 13.9511) knots 0 0 0 0 0.018093 0.034604 0.034604 0.034604 0.034604
  spline S39 degree 3 poles (0.56, 13.9511) (0.5225, 13.9104) (0.4445, 13.8259) (0.3351, 13.7902) (0.2783, 13.7717) knots 0 0 0 0 0.016316 0.033898 0.033898 0.033898 0.033898
  spline S40 degree 3 poles (0.2783, 13.7717) (0.325, 13.7523) (0.4126, 13.716) (0.4754, 13.6451) (0.5048, 13.612) knots 0 0 0 0 0.014933 0.028029 0.028029 0.028029 0.028029
  spline S41 degree 3 poles (0.5048, 13.612) (0.5263, 13.575) (0.5707, 13.4983) (0.5758, 13.4096) (0.5784, 13.3638) knots 0 0 0 0 0.012661 0.026224 0.026224 0.026224 0.026224
  spline S42 degree 3 poles (0.5784, 13.3638) (0.572, 13.294) (0.5591, 13.1548) (0.4673, 13.0493) (0.4216, 12.9968) knots 0 0 0 0 0.020468 0.040823 0.040823 0.040823 0.040823
  spline S43 degree 3 poles (0.4216, 12.9968) (0.3629, 12.9534) (0.2391, 12.862) (0.0851, 12.8529) (0.0041, 12.8481) knots 0 0 0 0 0.021415 0.045172 0.045172 0.045172 0.045172
  spline S44 degree 3 poles (0.0041, 12.8481) (-0.0775, 12.8531) (-0.2333, 12.8627) (-0.3581, 12.9558) (-0.4175, 13.0002) knots 0 0 0 0 0.02394 0.045691 0.045691 0.045691 0.045691
  spline S45 degree 3 poles (-0.4175, 13.0002) (-0.464, 13.0535) (-0.5569, 13.1599) (-0.5704, 13.3005) (-0.5771, 13.3706) knots 0 0 0 0 0.020682 0.041247 0.041247 0.041247 0.041247
  spline S46 degree 3 poles (-0.5771, 13.3706) (-0.5744, 13.415) (-0.5691, 13.5015) (-0.5254, 13.5763) (-0.5041, 13.6127) knots 0 0 0 0 0.013139 0.025609 0.025609 0.025609 0.025609
  spline S47 degree 3 poles (-0.5041, 13.6127) (-0.4752, 13.6456) (-0.4138, 13.7156) (-0.3279, 13.7522) (-0.2824, 13.7717) knots 0 0 0 0 0.012951 0.027588 0.027588 0.027588 0.027588
  spline S48 degree 3 poles (-0.2824, 13.7717) (-0.3393, 13.7937) (-0.4485, 13.8359) (-0.5258, 13.9235) (-0.5628, 13.9654) knots 0 0 0 0 0.018015 0.034524 0.034524 0.034524 0.034524
  spline S49 degree 3 poles (-0.5628, 13.9654) (-0.5908, 14.013) (-0.6487, 14.1115) (-0.6555, 14.2257) (-0.6589, 14.2846) knots 0 0 0 0 0.016344 0.033768 0.033768 0.033768 0.033768
  spline S50 degree 3 poles (-0.6589, 14.2846) (-0.6515, 14.3666) (-0.6368, 14.5296) (-0.5304, 14.6539) (-0.4775, 14.7157) knots 0 0 0 0 0.024034 0.04782 0.04782 0.04782 0.04782
  spline S51 degree 3 poles (-0.4775, 14.7157) (-0.4102, 14.7666) (-0.2692, 14.8732) (-0.0924, 14.8845) (0, 14.8904) knots 0 0 0 0 0.024757 0.051851 0.051851 0.051851 0.051851
  spline S52 degree 3 poles (0, 14.8904) (0.0924, 14.8844) (0.2694, 14.8731) (0.4102, 14.7662) (0.4775, 14.715) knots 0 0 0 0 0.027096 0.051881 0.051881 0.051881 0.051881
  spline S53 degree 3 poles (0.4775, 14.715) (0.5304, 14.6526) (0.6374, 14.5262) (0.6517, 14.3612) (0.6589, 14.2778) knots 0 0 0 0 0.02394 0.048393 0.048393 0.048393 0.048393
  spline S54 degree 3 poles (4.6371, 13.6284) (4.5829, 13.5312) (4.48, 13.3469) (4.3472, 13.1828) (4.2845, 13.1052) knots 0 0 0 0 0.033323 0.063198 0.063198 0.063198 0.063198
  line L29 (4.2845, 13.1052) -> (5.264, 13.1052)
  line L30 (5.264, 13.1052) -> (5.264, 12.8692)
  line L31 (5.264, 12.8692) -> (3.9693, 12.8692)
  line L32 (3.9693, 12.8692) -> (3.9693, 13.0602)
  spline S55 degree 3 poles (3.9693, 13.0602) (4.035, 13.1375) (4.178, 13.3057) (4.2883, 13.497) (4.3479, 13.6005) knots 0 0 0 0 0.030361 0.066089 0.066089 0.066089 0.066089
  spline S56 degree 3 poles (4.3479, 13.6005) (4.4067, 13.713) (4.5231, 13.9357) (4.5998, 14.175) (4.6378, 14.2935) knots 0 0 0 0 0.038005 0.075246 0.075246 0.075246 0.075246
  spline S57 degree 3 poles (4.6378, 14.2935) (4.6603, 14.3807) (4.7067, 14.5614) (4.7234, 14.7472) (4.7319, 14.8433) knots 0 0 0 0 0.02698 0.055862 0.055862 0.055862 0.055862
  line L33 (4.7319, 14.8433) -> (4.9843, 14.8433)
  spline S58 degree 3 poles (4.9843, 14.8433) (4.9782, 14.7561) (4.9647, 14.5633) (4.9174, 14.3757) (4.8916, 14.273) knots 0 0 0 0 0.026179 0.057876 0.057876 0.057876 0.057876
  spline S59 degree 3 poles (4.8916, 14.273) (4.8587, 14.1624) (4.7926, 13.9401) (4.6891, 13.7326) (4.6371, 13.6284) knots 0 0 0 0 0.034557 0.069417 0.069417 0.069417 0.069417
  spline S60 degree 3 poles (-4.558, 14.8904) (-4.4847, 14.886) (-4.3446, 14.8778) (-4.2295, 14.798) (-4.1746, 14.7601) knots 0 0 0 0 0.021564 0.041189 0.041189 0.041189 0.041189
  spline S61 degree 3 poles (-4.1746, 14.7601) (-4.1298, 14.7104) (-4.0354, 14.6057) (-4.0095, 14.4668) (-3.9959, 14.3938) knots 0 0 0 0 0.01968 0.041471 0.041471 0.041471 0.041471
  line L34 (-3.9959, 14.3938) -> (-4.2319, 14.3719)
  spline S62 degree 3 poles (-4.2319, 14.3719) (-4.2424, 14.4218) (-4.2613, 14.5119) (-4.3202, 14.5821) (-4.3465, 14.6134) knots 0 0 0 0 0.015008 0.027097 0.027097 0.027097 0.027097
  spline S63 degree 3 poles (-4.3465, 14.6134) (-4.3776, 14.6353) (-4.4426, 14.681) (-4.522, 14.6859) (-4.5635, 14.6884) knots 0 0 0 0 0.011173 0.023358 0.023358 0.023358 0.023358
  spline S64 degree 3 poles (-4.5635, 14.6884) (-4.5995, 14.6866) (-4.6693, 14.683) (-4.7318, 14.6517) (-4.762, 14.6366) knots 0 0 0 0 0.010703 0.020715 0.020715 0.020715 0.020715
  spline S65 degree 3 poles (-4.762, 14.6366) (-4.7892, 14.6178) (-4.8439, 14.5799) (-4.8824, 14.5255) (-4.9018, 14.4981) knots 0 0 0 0 0.009841 0.019815 0.019815 0.019815 0.019815
  spline S66 degree 3 poles (-4.9018, 14.4981) (-4.9197, 14.4647) (-4.9596, 14.3904) (-4.9813, 14.3089) (-4.9932, 14.2642) knots 0 0 0 0 0.011348 0.025194 0.025194 0.025194 0.025194
  spline S67 degree 3 poles (-4.9932, 14.2642) (-5.0039, 14.2148) (-5.0255, 14.1159) (-5.0285, 14.0147) (-5.03, 13.964) knots 0 0 0 0 0.015125 0.030296 0.030296 0.030296 0.030296
  spline S68 degree 3 poles (-5.03, 13.964) (-5.0299, 13.9572) (-5.0297, 13.9408) (-5.0291, 13.9245) (-5.0287, 13.9149) knots 0 0 0 0 0.002047 0.004913 0.004913 0.004913 0.004913
  spline S69 degree 3 poles (-5.0287, 13.9149) (-5.0016, 13.9524) (-4.9465, 14.0284) (-4.8675, 14.0794) (-4.8274, 14.1052) knots 0 0 0 0 0.013741 0.027912 0.027912 0.027912 0.027912
  spline S70 degree 3 poles (-4.8274, 14.1052) (-4.784, 14.1265) (-4.6967, 14.1692) (-4.5998, 14.1752) (-4.5512, 14.1782) knots 0 0 0 0 0.014368 0.028825 0.028825 0.028825 0.028825
  spline S71 degree 3 poles (-4.5512, 14.1782) (-4.4716, 14.1707) (-4.3123, 14.1556) (-4.1914, 14.0507) (-4.131, 13.9981) knots 0 0 0 0 0.023357 0.04675 0.04675 0.04675 0.04675
  spline S72 degree 3 poles (-4.131, 13.9981) (-4.0809, 13.9312) (-3.9757, 13.7908) (-3.9648, 13.6153) (-3.9591, 13.5234) knots 0 0 0 0 0.024534 0.051481 0.051481 0.051481 0.051481
  spline S73 degree 3 poles (-3.9591, 13.5234) (-3.9651, 13.4285) (-3.9766, 13.247) (-4.0862, 13.1025) (-4.1385, 13.0336) knots 0 0 0 0 0.02782 0.053201 0.053201 0.053201 0.053201
  spline S74 degree 3 poles (-4.1385, 13.0336) (-4.2026, 12.9795) (-4.3326, 12.8699) (-4.5022, 12.8554) (-4.588, 12.8481) knots 0 0 0 0 0.024536 0.049711 0.049711 0.049711 0.049711
  spline S75 degree 3 poles (-4.588, 12.8481) (-4.6516, 12.8524) (-4.7783, 12.861) (-4.8894, 12.9225) (-4.9448, 12.9531) knots 0 0 0 0 0.018857 0.037596 0.037596 0.037596 0.037596
  spline S76 degree 3 poles (-4.9448, 12.9531) (-4.9957, 12.9926) (-5.1003, 13.0737) (-5.1598, 13.192) (-5.1903, 13.2526) knots 0 0 0 0 0.019093 0.039165 0.039165 0.039165 0.039165
  spline S77 degree 3 poles (-5.1903, 13.2526) (-5.2147, 13.3313) (-5.2713, 13.5142) (-5.2732, 13.7061) (-5.2742, 13.8153) knots 0 0 0 0 0.024607 0.057161 0.057161 0.057161 0.057161
  spline S78 degree 3 poles (-5.2742, 13.8153) (-5.2727, 13.9309) (-5.2699, 14.138) (-5.2152, 14.3376) (-5.191, 14.4258) knots 0 0 0 0 0.034493 0.061835 0.061835 0.061835 0.061835
  spline S79 degree 3 poles (-5.191, 14.4258) (-5.1613, 14.496) (-5.1045, 14.63) (-4.9954, 14.7259) (-4.9434, 14.7717) knots 0 0 0 0 0.022523 0.043023 0.043023 0.043023 0.043023
  spline S80 degree 3 poles (-4.9434, 14.7717) (-4.8854, 14.8063) (-4.7667, 14.8771) (-4.6286, 14.8859) (-4.558, 14.8904) knots 0 0 0 0 0.019951 0.040848 0.040848 0.040848 0.040848
  spline S81 degree 3 poles (0.0205, 18.3392) (0.1058, 18.3341) (0.2688, 18.3244) (0.4022, 18.231) (0.4659, 18.1864) knots 0 0 0 0 0.025071 0.047918 0.047918 0.047918 0.047918
  spline S82 degree 3 poles (0.4659, 18.1864) (0.5173, 18.1303) (0.6231, 18.0149) (0.6495, 17.8605) (0.663, 17.7812) knots 0 0 0 0 0.022351 0.045918 0.045918 0.045918 0.045918
  line L35 (0.663, 17.7812) -> (0.4052, 17.7594)
  spline S83 degree 3 poles (0.4052, 17.7594) (0.3941, 17.8167) (0.3736, 17.9227) (0.3041, 18.0048) (0.2722, 18.0425) knots 0 0 0 0 0.017163 0.031746 0.031746 0.031746 0.031746
  spline S84 degree 3 poles (0.2722, 18.0425) (0.2353, 18.0701) (0.1606, 18.1261) (0.0676, 18.1335) (0.0205, 18.1373) knots 0 0 0 0 0.01353 0.027394 0.027394 0.027394 0.027394
  spline S85 degree 3 poles (0.0205, 18.1373) (-0.0365, 18.1316) (-0.1512, 18.1201) (-0.2367, 18.0426) (-0.2797, 18.0036) knots 0 0 0 0 0.016709 0.03364 0.03364 0.03364 0.03364
  spline S86 degree 3 poles (-0.2797, 18.0036) (-0.3155, 17.9536) (-0.3911, 17.8478) (-0.3985, 17.7176) (-0.4025, 17.6489) knots 0 0 0 0 0.018074 0.038228 0.038228 0.038228 0.038228
  spline S87 degree 3 poles (-0.4025, 17.6489) (-0.3988, 17.584) (-0.392, 17.4614) (-0.3188, 17.3634) (-0.2844, 17.3174) knots 0 0 0 0 0.019023 0.03589 0.03589 0.03589 0.03589
  spline S88 degree 3 poles (-0.2844, 17.3174) (-0.2411, 17.282) (-0.1512, 17.2087) (-0.0353, 17.2003) (0.0246, 17.196) knots 0 0 0 0 0.016388 0.033928 0.033928 0.033928 0.033928
  spline S89 degree 3 poles (0.0246, 17.196) (0.0628, 17.198) (0.1378, 17.202) (0.2056, 17.2341) (0.2387, 17.2499) knots 0 0 0 0 0.011369 0.022275 0.022275 0.022275 0.022275
  spline S90 degree 3 poles (0.2387, 17.2499) (0.2687, 17.2689) (0.3274, 17.3062) (0.3686, 17.3622) (0.3888, 17.3897) knots 0 0 0 0 0.010537 0.020672 0.020672 0.020672 0.020672
  line L36 (0.3888, 17.3897) -> (0.6194, 17.3597)
  line L37 (0.6194, 17.3597) -> (0.4256, 16.3324)
  line L38 (0.4256, 16.3324) -> (-0.5689, 16.3324)
  line L39 (-0.5689, 16.3324) -> (-0.5689, 16.567)
  line L40 (-0.5689, 16.567) -> (0.2292, 16.567)
  line L41 (0.2292, 16.567) -> (0.337, 17.1046)
  spline S91 degree 3 poles (0.337, 17.1046) (0.2772, 17.068) (0.1608, 16.9967) (0.0251, 16.9848) (-0.0409, 16.9791) knots 0 0 0 0 0.020714 0.040305 0.040305 0.040305 0.040305
  spline S92 degree 3 poles (-0.0409, 16.9791) (-0.1246, 16.9864) (-0.2909, 17.001) (-0.4192, 17.1076) (-0.4829, 17.1605) knots 0 0 0 0 0.02457 0.048806 0.048806 0.048806 0.048806